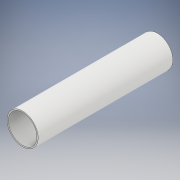
# Autodesk Inventor part: 2inpvc_pipe
Saved by Autodesk Inventor 2018 (Build 220112000, 112)
## iProperties
Created: 2018-09-09
Part Number: 2inpvc_pipe
Material: Generic
Document SubType Name: Modeling
Designer: Fredy Espana C
Density: 1 g/cm^3
Appearance: Default
Author: Fredy Espana C
Autodesk Inventor part; units mm, degrees
ref_plane "YZ Plane" through (0, 0, 0) normal (1, 0, 0) x (0, 1, 0)
ref_plane "XZ Plane" through (0, 0, 0) normal (0, 1, 0) x (-1, 0, 0)
ref_plane "XY Plane" through (0, 0, 0) normal (0, 0, 1) x (1, 0, 0)
sketch "Sketch1" plane through (0, 0, 0) normal (0, 0, 1) x (1, 0, 0)
  circle A0 centre (0, 0) radius 25.4
  circle A1 centre (0, 0) radius 23.4
  dimension "d0" = 50.8
  dimension "d1" = 2
  constraints: 2 centre point, 1 coincident, 1 concentric
  measures "d0" diameter of A0
  measures "d1" radial gap between concentric circles of A0 A1
extrude "Extrusion1" add sketch "Sketch1" along normal blind 220
body "Solid1"
